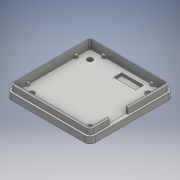
# Autodesk Inventor part: MyNavX_Mini_Base
Saved by Autodesk Inventor 2016 (Build 200138000, 138)
## iProperties
Created: 2016-12-19
Part Number: MyNavX_Mini_Base
Material: Generic
Document SubType Name: Modeling
Designer: Applefamily
Density: 1 g/cm^3
Appearance: Default
Author: Applefamily
Autodesk Inventor part; units mm, degrees
ref_plane "YZ Plane" through (0, 0, 0) normal (1, 0, 0) x (0, 1, 0)
ref_plane "XZ Plane" through (0, 0, 0) normal (0, 1, 0) x (-1, 0, 0)
ref_plane "XY Plane" through (0, 0, 0) normal (0, 0, 1) x (1, 0, 0)
sketch "Sketch1" plane through (0, 0, 0) normal (0, 0, 1) x (1, 0, 0)
  line L0 (-20.5, 23.5) -> (20.5, 23.5)
  line L1 (23.5, 20.5) -> (23.5, -20.5)
  line L2 (20.5, -23.5) -> (-20.5, -23.5)
  line L3 (-23.5, -20.5) -> (-23.5, 20.5)
  arc A0 (-20.5, 23.5) -> (-23.5, 20.5) centre (-20.5, 20.5) ccw
  arc A1 (23.5, 20.5) -> (20.5, 23.5) centre (20.5, 20.5) ccw
  arc A2 (20.5, -23.5) -> (23.5, -20.5) centre (20.5, -20.5) ccw
  arc A3 (-23.5, -20.5) -> (-20.5, -23.5) centre (-20.5, -20.5) ccw
  point P0 (0, 0)
  point P1 (-23.5, 23.5)
  point P2 (23.5, 23.5)
  point P3 (-23.5, -23.5)
  point P4 (23.5, 0)
  point P5 (0, 23.5)
  dimension "d0" = 47
  dimension "d1" = 47
  dimension "d2" = 3
  dimension "d3" = 3
  constraints: 8 end point, 8 point on circle, 8 tangent, 6 point on line, 4 centre point, 2 equal radius, 2 midpoint, 2 parallel, 1 horizontal, 1 horizontal alignment, 1 perpendicular, 1 vertical alignment
  measures "d0" distance of point (-23.5, -23.5) point (-23.5, 23.5)
  measures "d1" distance of point (-23.5, 23.5) point (23.5, 23.5)
  measures "d2" radius of A0
  measures "d3" radius of A1
extrude "Extrusion1" add sketch "Sketch1" along normal blind 2
sketch "Sketch2" plane through (0, 0, 2) normal (0, 0, 1) x (1, 0, 0)
  line L0 (-1, 18.75) -> (11.25, 18.75)
  line L1 (11.25, 18.75) -> (11.25, 14.25)
  line L2 (11.25, 14.25) -> (-1, 14.25)
  line L3 (-1, 14.25) -> (-1, 18.75)
  line L4 (23.5, -20.5) -> (23.5, 20.5) projected
  line L5 (-20.5, -23.5) -> (20.5, -23.5) projected
  point P0 (0, 0)
  dimension "d6" = 12.25
  dimension "d7" = 12.25
  dimension "d8" = 4.5
  dimension "d9" = 37.75
  constraints: 8 end point, 2 parallel, 1 horizontal, 1 perpendicular
  measures "d6" distance between parallel lines of L4 L1
  measures "d7" distance of L0.start L0.end
  measures "d8" distance of L0.end L1.end
  measures "d9" distance between parallel lines of L5 L2
extrude "Extrusion2" cut sketch "Sketch2" against normal blind 1.5
sketch "Sketch3" plane through (0, 0, 2) normal (0, 0, 1) x (1, 0, 0)
  line L0 (-1, 14.25) -> (-1, 18.75) projected
  line L1 (-1, 18.75) -> (11.25, 18.75) projected
  line L2 (11.25, 18.75) -> (11.25, 14.25) projected
  line L3 (11.25, 14.25) -> (-1, 14.25) projected
  line L4 (20.5, 23.5) -> (-20.5, 23.5) projected
  arc A0 (-20.5, 23.5) -> (-23.5, 20.5) centre (-20.5, 20.5) ccw projected
  line L5 (-23.5, 20.5) -> (-23.5, -20.5) projected
  arc A1 (-23.5, -20.5) -> (-20.5, -23.5) centre (-20.5, -20.5) ccw projected
  line L6 (-20.5, -23.5) -> (20.5, -23.5) projected
  arc A2 (20.5, -23.5) -> (23.5, -20.5) centre (20.5, -20.5) ccw projected
  line L7 (23.5, -20.5) -> (23.5, 20.5) projected
  arc A3 (23.5, 20.5) -> (20.5, 23.5) centre (20.5, 20.5) ccw projected
  line L8 (-21.5, -20.5) -> (-21.5, 20.5)
  arc A4 (-20.5, 21.5) -> (-21.5, 20.5) centre (-20.5, 20.5) ccw
  line L9 (-20.5, 21.5) -> (20.5, 21.5)
  arc A5 (21.5, 20.5) -> (20.5, 21.5) centre (20.5, 20.5) ccw
  line L10 (21.5, 20.5) -> (21.5, -20.5)
  arc A6 (20.5, -21.5) -> (21.5, -20.5) centre (20.5, -20.5) ccw
  line L11 (20.5, -21.5) -> (-20.5, -21.5)
  arc A7 (-21.5, -20.5) -> (-20.5, -21.5) centre (-20.5, -20.5) ccw
  point P0 (0, 0)
  dimension "d12" = 2
  constraints: 8 end point, 8 point on circle, 4 centre point, 7 other
  measures "d12" distance between parallel lines of L5 L8
extrude "Extrusion3" add sketch "Sketch3" along normal blind 1.5 contours A3 L7 A2 L6 A1 L5 A0 L4
sketch "Sketch5" plane through (0, 0, 3.5) normal (0, 0, 1) x (1, 0, 0)
  line L0 (-21.5, -20.5) -> (-21.5, 20.5) projected
  arc A0 (-20.5, 21.5) -> (-21.5, 20.5) centre (-20.5, 20.5) ccw projected
  arc A1 (-20.5, 21.5) -> (-21.5, 20.5) centre (-20.5, 20.5) ccw projected
  line L1 (-21.5, 20.5) -> (-21.5, -20.5) projected
  arc A2 (-21.5, -20.5) -> (-20.5, -21.5) centre (-20.5, -20.5) ccw projected
  line L2 (-20.5, -21.5) -> (20.5, -21.5) projected
  arc A3 (20.5, -21.5) -> (21.5, -20.5) centre (20.5, -20.5) ccw projected
  line L3 (21.5, -20.5) -> (21.5, 20.5) projected
  arc A4 (21.5, 20.5) -> (20.5, 21.5) centre (20.5, 20.5) ccw projected
  line L4 (20.5, 21.5) -> (-20.5, 21.5) projected
  line L5 (-1, 14.25) -> (-1, 18.75) projected
  line L6 (-1, 18.75) -> (11.25, 18.75) projected
  line L7 (11.25, 18.75) -> (11.25, 14.25) projected
  line L8 (11.25, 14.25) -> (-1, 14.25) projected
  arc A5 (-20.5, 22.4) -> (-22.4, 20.5) centre (-20.5, 20.5) ccw
  line L9 (-22.4, 20.5) -> (-22.4, -20.5)
  arc A6 (-22.4, -20.5) -> (-20.5, -22.4) centre (-20.5, -20.5) ccw
  line L10 (-20.5, -22.4) -> (20.5, -22.4)
  arc A7 (20.5, -22.4) -> (22.4, -20.5) centre (20.5, -20.5) ccw
  arc A8 (22.4, 20.5) -> (20.5, 22.4) centre (20.5, 20.5) ccw
  line L11 (20.5, 22.4) -> (-20.5, 22.4)
  line L12 (21.5, -11.75) -> (22.4, -11.75)
  line L13 (-20.5, -23.5) -> (20.5, -23.5) projected
  line L14 (21.5, -20.5) -> (21.5, 20.5) projected
  line L15 (21.5, -1.25) -> (22.4, -1.25)
  line L16 (22.4, -20.5) -> (22.4, -11.75)
  line L17 (22.4, -1.25) -> (22.4, 20.5)
  arc A9 (-20.5, 21.5) -> (-21.5, 20.5) centre (-20.5, 20.5) ccw projected
  line L18 (-20.5, 21.5) -> (20.5, 21.5) projected
  arc A10 (21.5, 20.5) -> (20.5, 21.5) centre (20.5, 20.5) ccw projected
  line L19 (21.5, 20.5) -> (21.5, -20.5) projected
  arc A11 (20.5, -21.5) -> (21.5, -20.5) centre (20.5, -20.5) ccw projected
  line L20 (20.5, -21.5) -> (-20.5, -21.5) projected
  arc A12 (-21.5, -20.5) -> (-20.5, -21.5) centre (-20.5, -20.5) ccw projected
  line L21 (-21.5, -20.5) -> (-21.5, 20.5) projected
  line L22 (20.5, 23.5) -> (-20.5, 23.5) projected
  arc A13 (-20.5, 23.5) -> (-23.5, 20.5) centre (-20.5, 20.5) ccw projected
  line L23 (-23.5, 20.5) -> (-23.5, -20.5) projected
  arc A14 (-23.5, -20.5) -> (-20.5, -23.5) centre (-20.5, -20.5) ccw projected
  line L24 (-20.5, -23.5) -> (20.5, -23.5) projected
  arc A15 (20.5, -23.5) -> (23.5, -20.5) centre (20.5, -20.5) ccw projected
  line L25 (23.5, -20.5) -> (23.5, 20.5) projected
  arc A16 (23.5, 20.5) -> (20.5, 23.5) centre (20.5, 20.5) ccw projected
  point P0 (0, 0)
  dimension "d24" = 0.9
  dimension "d25" = 11.75
  dimension "d26" = 10.5
  constraints: 14 end point, 8 point on circle, 4 centre point, 4 perpendicular, 2 point on line, 5 other
  measures "d24" distance between parallel lines of L4 L11
  measures "d25" distance between parallel lines of L13 L12
  measures "d26" distance between parallel lines of L15 L12
extrude "Extrusion5" add sketch "Sketch5" along normal blind 3.5 contours A2 L2 A3 L3 L12 L16 A7 L10 A6 L9 A5 L11 A8 L17 L15 A4 L4 A0 L0
chamfer "Chamfer1" distance 0.5 angle 45 9 edges at (22.4, 9.625, 7) (21.8435, 21.8435, 7) (0, 22.4, 7) (-21.8435, 21.8435, 7) (-22.4, 0, 7) (-21.8435, -21.8435, 7) (0, -22.4, 7) (21.8435, -21.8435, 7) (22.4, -16.125, 7)
sketch "Sketch4" plane through (0, 0, 2) normal (0, 0, 1) x (1, 0, 0)
  line L0 (-20.3, 20.3) -> (20.3, 20.3)
  line L1 (20.3, 20.3) -> (20.3, -20.3)
  line L2 (20.3, -20.3) -> (-20.3, -20.3)
  line L3 (-20.3, -20.3) -> (-20.3, 20.3)
  line L4 (21.5, -20.5) -> (21.5, 20.5) projected
  circle A0 centre (21.5, -13.5) radius 1.2
  line L5 (-21.5, -20.5) -> (-21.5, 20.5) projected
  circle A1 centre (-21.5, -13.5) radius 1.2
  line L6 (-20.5, -21.5) -> (20.5, -21.5) projected
  circle A2 centre (-13.5, -21.5) radius 1.2
  circle A3 centre (13.5, -21.5) radius 1.2
  line L7 (20.5, 21.5) -> (-20.5, 21.5) projected
  circle A4 centre (-13.5, 21.5) radius 1.2
  circle A5 centre (13.5, 21.5) radius 1.2
  circle A6 centre (-21.5, 13.5) radius 1.2
  circle A7 centre (21.5, 13.5) radius 1.2
  line L8 (-20.5, -23.5) -> (20.5, -23.5) projected
  line L9 (-23.5, 20.5) -> (-23.5, -20.5) projected
  line L10 (23.5, -20.5) -> (23.5, 20.5) projected
  line L11 (20.5, 23.5) -> (-20.5, 23.5) projected
  circle A8 centre (-16.25, 16.25) radius 1.5
  circle A9 centre (16.25, 16.25) radius 1.5
  circle A10 centre (-16.25, -16.25) radius 1.5
  circle A11 centre (16.25, -16.25) radius 1.5
  circle A12 centre (-16.25, 16.25) radius 3
  circle A13 centre (16.25, 16.25) radius 3
  circle A14 centre (16.25, -16.25) radius 3
  circle A15 centre (-16.25, -16.25) radius 3
  point P0 (0, 0)
  point P1 (-20.3, 0)
  point P2 (0, -20.3)
  dimension "d15" = 40.6
  dimension "d16" = 40.6
  dimension "d17" = 10
  dimension "d18" = 10
  dimension "d19" = 10
  dimension "d20" = 10
  dimension "d21" = 10
  dimension "d33" = 3
  dimension "d37" = 32.5
  dimension "d40" = 32.5
  dimension "d43" = 16.25
  dimension "d44" = 16.25
  dimension "d45" = 6
  dimension "d46" = 6
  dimension "d47" = 6
  dimension "d48" = 6
  constraints: 16 centre point, 8 end point, 8 point on line, 8 tangent, 4 coincident, 3 vertical alignment, 2 horizontal, 2 horizontal alignment, 2 midpoint, 2 parallel, 1 perpendicular, 1 vertical, 6 other
  measures "d15" distance of L0.start L0.end
  measures "d16" distance of L2.end L0.start
  measures "d17" distance from line of L8 A1.centre
  measures "d18" distance from line of L9 A2.centre
  measures "d19" distance from line of L10 A3.centre
  measures "d20" distance from line of L8 A0.centre
  measures "d21" distance from line of L11 A7.centre
  measures "d33" diameter of A8
  measures "d37" distance of A8.centre A9.centre
  measures "d40" distance of A8.centre A10.centre
  measures "d43" horizontal distance of point (0, 0) A8.centre
  measures "d44" horizontal distance of A8.centre point (0, 0)
  measures "d45" diameter of A12
  measures "d46" diameter of A13
  measures "d47" diameter of A14
  measures "d48" diameter of A15
extrude "Extrusion4" add sketch "Sketch4" along normal blind 1.5 contours A4 L7 | A6 L5 | A5 L7 | A4 L7 | A1 L5 | L5 A6 | A5 L7 | L5 A1 | A7 L4 | A2 L6 | A0 L4 | A7 L4 | A3 L6 | A2 L6 | A0 L4 | A3 L6
extrude "Extrusion6" cut sketch "Sketch4" against normal blind 3.5 contours A8 | A9 | A10 | A11
chamfer "Chamfer2" distance 0.25 angle 45 8 edges at (-20.3, -13.5, 3.5) (-20.3, 13.5, 3.5) (-13.5, 20.3, 3.5) (13.5, 20.3, 3.5) (20.3, 13.5, 3.5) (20.3, -13.5, 3.5) (13.5, -20.3, 3.5) (-13.5, -20.3, 3.5)
equation "\"d18\" = d17"
equation "\"d19\" = d18"
equation "\"d20\" = d19"
equation "\"d21\" = d20"
equation "\"d33\" = d32"
equation "\"d43\" = 0.5 * d40"
equation "\"d44\" = d43"
equation "\"d32\" = 3"
body "Solid1"
